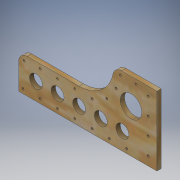
# Autodesk Inventor part: arm droit
Saved by Autodesk Inventor 2016 (Build 200138000, 138)
## iProperties
Created: 2016-01-30
Part Number: arm droit
Material: Generic
Document SubType Name: Modeling
Designer: ares-b02
Density: 1 g/cm^3
Appearance: Plywood - Weathered
Author: ares-b02
Autodesk Inventor part; units mm, degrees
ref_plane "YZ Plane" through (0, 0, 0) normal (1, 0, 0) x (0, 1, 0)
ref_plane "XZ Plane" through (0, 0, 0) normal (0, 1, 0) x (-1, 0, 0)
ref_plane "XY Plane" through (0, 0, 0) normal (0, 0, 1) x (1, 0, 0)
sketch "Sketch1" plane through (0, 0, 0) normal (0, 0, 1) x (1, 0, 0)
  line L0 (-175.7553, 1.949) -> (-175.7553, -36.151)
  line L1 (-175.7553, -36.151) -> (27.4447, -36.151)
  line L2 (27.4447, -36.151) -> (27.4447, 65.449)
  line L3 (27.4447, 65.449) -> (-36.0553, 65.449)
  line L4 (-163.0553, 14.649) -> (-86.8553, 14.649)
  line L5 (-36.0553, 65.449) -> (-36.0553, 65.449)
  arc A0 (-86.8553, 14.649) -> (-36.0553, 65.449) centre (-86.8553, 65.449) ccw
  arc A1 (-163.0553, 14.649) -> (-175.7553, 1.949) centre (-163.0553, 1.949) ccw
  point P0 (0, 0)
  point P1 (-175.7553, 14.649)
  dimension "d0" = 203.2
  dimension "d1" = 101.6
  dimension "d2" = 63.5
  dimension "d3" = 50.8
  dimension "d7" = 50.8
  dimension "d8" = 12.7
  constraints: 12 end point, 4 perpendicular, 4 point on circle, 4 tangent, 2 centre point, 2 point on line, 1 horizontal, 1 vertical
  measures "d0" distance of L0.end L1.end
  measures "d1" distance of L1.end L2.end
  measures "d2" distance of L2.end L3.end
  measures "d3" distance of point (-175.755, 14.649) L0.end
  measures "d7" radius of A0
  measures "d8" radius of A1
extrude "Extrusion1" add sketch "Sketch1" along normal blind 6.35
hole "Hole1" at (-169.4053, -29.801, 6.35) direction (0, 0, -1) diameter 3.175 end through all
pattern_linear "Rectangular Pattern1" count 7 spacing 25.4 along (1, 0, 0) of "Hole1"
hole "Hole2" at (-144.0053, 8.299, 6.35) direction (0, 0, -1) diameter 3.175 end through all
pattern_linear "Rectangular Pattern2" count 4 spacing 25.4 along (1, 0, 0) of "Hole2"
hole "Hole3" at (-46.2174, 19.2208, 6.35) direction (0, 0, -1) diameter 3.175 end through all
hole "Hole4" at (-32.5291, 39.1356, 6.35) direction (0, 0, -1) diameter 3.175 end through all
hole "Hole5" at (-26.0985, 59.099, 6.35) direction (0, 0, -1) diameter 3.175 end through all
pattern_linear "Rectangular Pattern3" count 2 spacing 22.86 along (1, 0, 0) of "Hole5"
hole "Hole6" at (-167.6661, 6.7836, 6.35) direction (0, 0, -1) diameter 3.175 end through all
fillet "Fillet1" radius 12.7 1 edges at (-36.0553, 65.449, 3.175)
hole "Hole7" at (-150.3553, -10.751, 6.35) direction (0, 0, -1) diameter 19.05 end through all
pattern_linear "Rectangular Pattern4" count 5 spacing 31.75 along (1, 0, 0) of "Hole7"
hole "Hole8" at (-10.6553, 27.349, 6.35) direction (0, 0, -1) diameter 31.75 end through all
hole "Hole9" at (14.7447, -23.451, 6.35) direction (0, 0, -1) diameter 3.175 end through all
pattern_linear "Rectangular Pattern5" count 4 spacing 25.4 along (0, 1, 0) of "Hole9"
body "Solid1"
